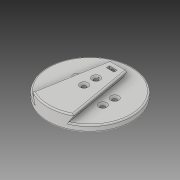
# Autodesk Inventor part: UR3_DoveTail_Interface_todevice
Saved by Autodesk Inventor 2017 SP1 (Build 210196100, 196)
## iProperties
Created: 2017-11-09
Part Number: UR3_DoveTail_Interface_todevice
Material: Generic
Document SubType Name: Modeling
Designer: Tomasz
Density: 1 g/cm^3
Appearance: Default
Author: Tomasz
Autodesk Inventor part; units mm, degrees
ref_plane "YZ Plane" through (0, 0, 0) normal (1, 0, 0) x (0, 1, 0)
ref_plane "XZ Plane" through (0, 0, 0) normal (0, 1, 0) x (-1, 0, 0)
sketch "Sketch1" plane through (0, 0, 0) normal (0, 1, 0) x (-1, 0, 0)
  circle A0 centre (0, 0) radius 31.5
  dimension "d0" = 63
  constraints: 1 centre point, 1 coincident
  measures "d0" diameter of A0
extrude "Extrusion1" add sketch "Sketch1" along normal blind 5
sketch "Sketch7" plane through (0, 5, 0) normal (0, 1, 0) x (1, 0, 0)
  circle A0 centre (0, 0) radius 31.5 projected
  circle A1 centre (0, 0) radius 31.5 projected
  line L0 (0, -31.5) -> (0, 31.5) construction
  line L1 (-13, -31.5) -> (13, -31.5)
  line L2 (-13, -31.5) -> (-3.6547, 21.5)
  line L3 (-3.6547, 21.5) -> (3.6547, 21.5)
  line L4 (3.6547, 21.5) -> (13, -31.5)
  line L5 (-13, -31.5) -> (-13, 27.1083) construction
  point P0 (0, 21.5)
  dimension "d26" = 26
  dimension "d27" = 53
  dimension "d28" = 10
  constraints: 12 end point, 4 point on circle, 3 midpoint, 2 horizontal, 2 vertical, 1 symmetric about line, 1 other
  measures "d26" distance of L1.start L1.end
  measures "d27" distance between parallel lines of L3 L1
  measures "d28" angle of L5 L2
ref_plane "Work Plane4" through (0, 0, 31.5) normal (0, 0, 1) x (1, 0, 0)
ref_plane "Work Plane5" through (0, 5, -21.5) normal (0, 0, 1) x (1, 0, 0)
sketch "Sketch8" plane through (0, 0, 31.5) normal (0, 0, 1) x (1, 0, 0)
  line L0 (-13, 5) -> (-16.4641, 11)
  line L1 (-16.4641, 11) -> (16.4641, 11)
  line L2 (16.4641, 11) -> (13, 5)
  line L3 (13, 5) -> (-13, 5)
  line L4 (31.5, 5) -> (-31.5, 5) projected
  line L5 (-13, 5) -> (13, 5)
  line L6 (0, 0) -> (0, 19.4313) construction
  dimension "d29" = 6
  dimension "d30" = 60
  constraints: 12 end point, 2 collinear, 1 symmetric about line, 1 vertical
  measures "d29" distance between parallel lines of L1 L3
  measures "d30" angle of L1 L0
sketch "Sketch9" plane through (0, 5, -21.5) normal (0, 0, 1) x (1, 0, 0)
  line L0 (0, -5) -> (0, 10.1177) construction
  line L1 (-3.6547, 0) -> (3.6547, 0)
  line L2 (-3.6547, 0) -> (-7.1188, 6)
  line L3 (-7.1188, 6) -> (7.1188, 6)
  line L4 (7.1188, 6) -> (3.6547, 0)
  dimension "d31" = 6
  dimension "d32" = 60
  constraints: 10 end point, 1 horizontal, 1 symmetric about line, 1 vertical
  measures "d31" distance between parallel lines of L1 L3
  measures "d32" angle of L2 L3
loft "Loft1" add profiles "Sketch8", "Sketch9"
sketch "Sketch10" plane through (0, 0, 0) normal (0, -1, 0) x (1, 0, 0)
  circle A0 centre (0, 0) radius 31.5 projected
  line L0 (-16.4641, 31.5) -> (-13, 31.5) projected
  circle A1 centre (0, 0) radius 35.5432
  constraints: 1 coincident, 3 other
extrude "Extrusion4" cut sketch "Sketch10" against normal up to surface (11 mm away)
ref_plane "Work Plane6" through (3.6547, 5, -17.5) normal (0, 0, -1) x (-1, 0, 0)
sketch "Sketch11" plane through (3.6547, 5, -17.5) normal (0, 0, -1) x (-1, 0, 0)
  line L0 (3.6547, -5) -> (3.6547, 5.9671) construction
  line L1 (16.1955, 0) -> (7.3093, 0) projected
  line L2 (7.3093, 0) -> (0, 0) projected
  line L3 (0, 0) -> (-8.8862, 0) projected
  line L4 (-8.8862, 0) -> (16.1955, 0) projected
  line L5 (6.5047, 1.8546) -> (3.6547, 0.2091)
  line L6 (3.6547, 0.2091) -> (0.8047, 1.8546)
  line L7 (0.8047, 1.8546) -> (0.8047, 5.1454)
  line L8 (0.8047, 5.1454) -> (3.6547, 6.7909)
  line L9 (3.6547, 6.7909) -> (6.5047, 5.1454)
  line L10 (6.5047, 5.1454) -> (6.5047, 1.8546)
  line L11 (0.8047, 5.1454) -> (0.8047, 6.7909)
  line L12 (0.8047, 6.7909) -> (6.5047, 6.7909)
  line L13 (6.5047, 6.7909) -> (6.5047, 5.1454)
  point P0 (3.6547, 3.5)
  dimension "d40" = 3.5
  dimension "d54" = 5.7
  constraints: 20 end point, 3 vertical, 1 collinear, 1 midpoint, 1 perpendicular, 1 point on line, 13 other
  measures "d40" distance from line of point (3.655, 3.5) L2
  measures "d54" distance between parallel lines of L10 L7
extrude "Extrusion5" cut sketch "Sketch11" against normal blind 2.4
sketch "Sketch12" plane through (3.6547, 5, -21.5) normal (0, 0, -1) x (-1, 0, 0)
  line L0 (3.6547, -5) -> (3.6547, 6) construction
  line L1 (0.8047, 6) -> (6.5047, 6) projected
  line L2 (16.1955, 0) -> (7.3093, 0) projected
  line L3 (7.3093, 0) -> (0, 0) projected
  line L4 (0, 0) -> (-8.8862, 0) projected
  line L5 (-8.8862, 0) -> (16.1955, 0) projected
  point P0 (-0.8937, 6)
  point P1 (6.0345, 6)
  point P2 (3.6547, 3.5)
  dimension "d44" = 3.5
  constraints: 2 end point, 1 midpoint, 1 point on line
  measures "d44" distance from line of L3 point (3.655, 3.5)
hole "Hole2" at (0, 8.5, -21.5) direction (0, 0, 1) diameter 3.5 depth 15
fillet "Fillet3" radius 1 7 edges at (11.4208, 11, 2.8978) (8.1376, 11, 30.4307) (-8.1376, 11, 30.4307) (-11.4208, 11, 2.8978) (5.3867, 8, -21.5) (-5.3867, 8, -21.5) (0, 11, -21.5)
fillet "Fillet4" radius 1 11 edges at (0, 0, -31.5) (0, 0, 31.5) (31.3488, 5, -3.083) (25.6544, 5, -18.2785) (0, 5, -31.5) (-25.6544, 5, -18.2785) (-31.3488, 5, -3.083) (24.5194, 5, 19.775) (31.3488, 5, 3.083) (-31.3488, 5, 3.083) (-24.5194, 5, 19.775)
sketch "Sketch13" plane through (0, 11, 0) normal (0, 1, 0) x (1, 0, 0)
  line L0 (0, 20.7455) -> (0, -17.2545) construction
  line L1 (-7.5419, 0) -> (9.0343, 0) construction
  point P0 (0, 0)
  point P1 (0, 4.5)
  point P2 (0, -4.5)
  dimension "d55" = 9
  constraints: 4 end point, 4 point on line, 1 horizontal, 1 symmetric about line, 1 vertical
  measures "d55" distance of point (0, -4.5) point (0, 4.5)
hole "Hole3" at (0, 11, -4.5) at (0, 11, 4.5) direction (0, -1, 0) diameter 3.2 end through all countersink diameter 6 countersink angle 90
sketch "Sketch14" plane through (0, 5, 0) normal (0, 1, 0) x (1, 0, 0)
  line L0 (-27, 0) -> (26.141, 0) construction
  line L1 (0, 24) -> (0, -21.4625) construction
  point P0 (0, 0)
  point P1 (-14, 4.5)
  point P2 (-14, -4.5)
  point P3 (14, 4.5)
  point P4 (14, -4.5)
  dimension "d63" = 9
  dimension "d64" = 28
  constraints: 4 end point, 4 symmetric about line, 2 point on line, 1 horizontal, 1 vertical
  measures "d63" distance of point (-14, -4.5) point (-14, 4.5)
  measures "d64" distance of point (14, 4.5) point (-14, 4.5)
hole "Hole4" at (-14, 5, -4.5) at (-14, 5, 4.5) at (14, 5, -4.5) at (14, 5, 4.5) direction (0, -1, 0) diameter 3.2 end through all countersink diameter 6 countersink angle 90
body "Solid1"
